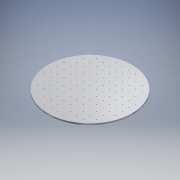
# Autodesk Inventor part: Circular_Breadboard
Saved by Autodesk Inventor 2016 (Build 200138000, 138)
## iProperties
Created: 2016-01-13
Part Number: Circular_Breadboard
Material: Aluminum 6061
Document SubType Name: Modeling
Designer: Conor Mow-Lowry
Density: 2.7 g/cm^3
Appearance: Aluminum - Flat
Mass: 11129.8 g
Surface Area: 6957.56 cm^2
Volume: 4122.15 cm^3
Author: Conor Mow-Lowry
Autodesk Inventor part; units mm, degrees
ref_plane "YZ Plane" through (0, 0, 0) normal (1, 0, 0) x (0, 1, 0)
ref_plane "XZ Plane" through (0, 0, 0) normal (0, 1, 0) x (-1, 0, 0)
ref_plane "XY Plane" through (0, 0, 0) normal (0, 0, 1) x (1, 0, 0)
sketch "Sketch1" plane through (0, 0, 0) normal (0, 1, 0) x (-1, 0, 0)
  circle A0 centre (0, 0) radius 322.5
  dimension "d0" = 645
  constraints: 1 centre point, 1 coincident
  measures "d0" diameter of A0
extrude "Extrusion1" add sketch "Sketch1" against normal blind 12.7
sketch "Sketch2" plane through (0, 0, 0) normal (0, 1, 0) x (1, 0, 0)
  circle A0 centre (0, 0) radius 322.5 projected
  line L0 (0, 322.5) -> (0, -322.5) construction
  line L1 (-322.5, 0) -> (322.5, 0) construction
  point P0 (25, -25)
  point P1 (25, -75)
  point P2 (25, -125)
  point P3 (25, -175)
  point P4 (25, -225)
  point P5 (25, -275)
  point P6 (75, -25)
  point P7 (75, -75)
  point P8 (75, -125)
  point P9 (75, -175)
  point P10 (75, -225)
  point P11 (75, -275)
  point P12 (125, -25)
  point P13 (175, -25)
  point P14 (225, -25)
  point P15 (125, -75)
  point P16 (175, -75)
  point P17 (225, -75)
  point P18 (125, -125)
  point P19 (175, -125)
  point P20 (225, -125)
  point P21 (275, -25)
  point P22 (275, -75)
  point P23 (125, -175)
  point P24 (175, -175)
  point P25 (225, -175)
  point P26 (125, -225)
  point P27 (175, -225)
  dimension "d3" = 25
  dimension "d4" = 25
  dimension "d7" = 50
  dimension "d10" = 50
  dimension "d13" = 50
  dimension "d16" = 50
  dimension "d19" = 50
  dimension "d22" = 50
  constraints: 8 horizontal alignment, 6 vertical alignment, 4 end point, 4 midpoint, 4 point on circle, 3 vertical, 2 horizontal, 1 perpendicular, 19 other
  measures "d3" distance from line of L1 point (25, -25)
  measures "d4" distance from line of L0 point (25, -25)
  measures "d7" distance of point (25, -25) point (25, -75)
  measures "d10" distance of point (25, -25) point (75, -25)
  measures "d13" distance of point (75, -25) point (125, -25)
  measures "d16" distance of point (125, -25) point (175, -25)
  measures "d19" distance of point (125, -25) point (125, -75)
  measures "d22" distance of point (275, -25) point (225, -25)
hole "Hole1" at (175, 0, 225) at (125, 0, 225) at (225, 0, 175) at (175, 0, 175) at (125, 0, 175) at (275, 0, 75) at (275, 0, 25) at (225, 0, 125) at (175, 0, 125) at (125, 0, 125) at (225, 0, 75) at (175, 0, 75) at (125, 0, 75) at (225, 0, 25) at (175, 0, 25) at (125, 0, 25) at (75, 0, 275) at (75, 0, 225) at (75, 0, 175) at (75, 0, 125) at (75, 0, 75) at (75, 0, 25) at (25, 0, 275) at (25, 0, 225) at (25, 0, 175) at (25, 0, 125) at (25, 0, 75) at (25, 0, 25) direction (0, -1, 0) diameter 4.917 end through all thread size "M6x1" class "6H" standard "ANSI Metric M Profile"
mirror "Mirror1" about plane through (0, 0, 0) normal (1, 0, 0) of "Hole1"
mirror "Mirror2" about plane through (0, 0, 0) normal (0, 0, 1) of "Hole1", "Mirror1"
chamfer "Chamfer1" distance 0.5 angle 45 2 edges at (322.5, 0, 0) (322.5, -12.7, 0)
equation "\"d3\" = 0.5 * x"
equation "\"d4\" = 0.5 * x"
equation "\"d7\" = x"
equation "\"d10\" = x"
equation "\"d13\" = x"
equation "\"d16\" = x"
equation "\"d19\" = x"
equation "\"d22\" = x"
equation "\"x\" = 50"
body "Solid1"
